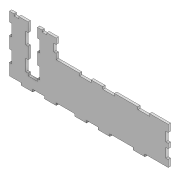
# Autodesk Inventor part: Frontal
Saved by Autodesk Inventor 2022 (Build 260153000, 153)
## iProperties
Created: 2022-06-21
Part Number: Frontal
Material: Generic
Document SubType Name: Modeling
Designer: ADMIN
Density: 1 g/cm^3
Appearance: Default
Author: ADMIN
Autodesk Inventor part; units mm, degrees
ref_plane "YZ Plane" through (0, 0, 0) normal (1, 0, 0) x (0, 1, 0)
ref_plane "XZ Plane" through (0, 0, 0) normal (0, 1, 0) x (-1, 0, 0)
ref_plane "XY Plane" through (0, 0, 0) normal (0, 0, 1) x (1, 0, 0)
sketch "Sketch1" plane through (0, 0, 0) normal (0, 0, 1) x (1, 0, 0)
  line L0 (-188.4506, 42.0684) -> (-148.4506, 42.0684)
  line L1 (-148.4506, 42.0684) -> (-148.4506, 2.0684)
  line L2 (-148.4506, 2.0684) -> (91.5494, 2.0684)
  line L3 (-198.4506, -77.9316) -> (91.5494, -77.9316)
  line L4 (91.5494, -77.9316) -> (91.5494, 2.0684)
  line L5 (-188.4506, -57.9316) -> (-208.4506, -57.9316)
  line L6 (-208.4506, -57.9316) -> (-208.4506, 42.0684)
  line L7 (-208.4506, 42.0684) -> (-248.4506, 42.0684)
  line L8 (-248.4506, 42.0684) -> (-248.4506, -77.9316)
  line L9 (-248.4506, -77.9316) -> (-198.4506, -77.9316)
  line L10 (-188.4506, -57.9316) -> (-188.4506, 42.0684)
  point P0 (0, 0)
  dimension "d2" = 80
  dimension "d3" = 40
  dimension "d23" = 40
  dimension "d24" = 20
  dimension "d26" = 20
  dimension "d27" = 120
  dimension "d28" = 120
  dimension "d58" = 280
  constraints: 22 end point, 3 perpendicular, 1 collinear, 1 horizontal, 1 vertical
  measures "d2" distance of L3.end L2.end
  measures "d3" distance of L0.start L0.end
  measures "d23" distance of L6.end L7.end
  measures "d24" distance of L5.start L5.end
  measures "d26" distance between parallel lines of L9 L5
  measures "d27" distance between parallel lines of L9 L7
  measures "d28" distance between parallel lines of L3 L0
  measures "d58" distance between parallel lines of L10 L4
extrude "Extrusion1" add sketch "Sketch1" along normal blind 5
sketch "Sketch2" plane through (0, 0, 5) normal (0, 0, 1) x (1, 0, 0)
  line L0 (91.5494, 2.0684) -> (-148.4506, 2.0684) projected
  line L1 (-148.4506, 2.0684) -> (-148.4506, 42.0684) projected
  line L2 (-148.4506, 42.0684) -> (-188.4506, 42.0684) projected
  line L3 (-248.4506, -77.9316) -> (91.5494, -77.9316) projected
  line L4 (91.5494, -77.9316) -> (91.5494, 2.0684) projected
  line L5 (91.5494, 2.0684) -> (-148.4506, 2.0684) projected
  line L6 (-98.4506, 2.0684) -> (-73.4506, 2.0684)
  line L7 (-73.4506, 2.0684) -> (-73.4506, -2.9316)
  line L8 (-73.4506, -2.9316) -> (-98.4506, -2.9316)
  line L9 (-98.4506, -2.9316) -> (-98.4506, 2.0684)
  line L10 (-48.4506, 2.0684) -> (-23.4506, 2.0684)
  line L11 (-23.4506, 2.0684) -> (-23.4506, -2.9316)
  line L12 (-23.4506, -2.9316) -> (-48.4506, -2.9316)
  line L13 (-48.4506, -2.9316) -> (-48.4506, 2.0684)
  line L14 (26.5494, 2.0684) -> (51.5494, 2.0684)
  line L15 (51.5494, 2.0684) -> (51.5494, -2.9316)
  line L16 (51.5494, -2.9316) -> (26.5494, -2.9316)
  line L17 (26.5494, -2.9316) -> (26.5494, 2.0684)
  line L18 (-148.4506, 42.0684) -> (-188.4506, 42.0684) projected
  line L19 (91.5494, -77.9316) -> (91.5494, 2.0684) projected
  line L20 (-73.4506, -7.9316) -> (-73.4506, -2.9316)
  line L21 (-98.4506, -2.9316) -> (-98.4506, -7.9316)
  line L22 (-23.4506, -7.9316) -> (-23.4506, -2.9316)
  line L23 (-48.4506, -2.9316) -> (-48.4506, -7.9316)
  line L24 (51.5494, -7.9316) -> (51.5494, -2.9316)
  line L25 (26.5494, -2.9316) -> (26.5494, -7.9316)
  line L26 (41.5494, -77.9316) -> (41.5494, -72.9316)
  line L27 (41.5494, -72.9316) -> (16.5494, -72.9316)
  line L28 (16.5494, -72.9316) -> (16.5494, -77.9316)
  line L29 (16.5494, -72.9316) -> (16.5494, -67.9316)
  line L30 (41.5494, -67.9316) -> (41.5494, -72.9316)
  line L31 (-188.4506, -57.9316) -> (-208.4506, -57.9316) projected
  line L32 (-208.4506, -57.9316) -> (-208.4506, 42.0684) projected
  line L33 (-208.4506, 42.0684) -> (-248.4506, 42.0684) projected
  line L34 (-248.4506, 42.0684) -> (-248.4506, -77.9316) projected
  line L35 (-188.4506, 42.0684) -> (-188.4506, -57.9316) projected
  line L36 (-208.4506, 42.0684) -> (-248.4506, 42.0684) projected
  line L37 (-238.4506, 42.0684) -> (-228.4506, 42.0684)
  line L38 (-228.4506, 42.0684) -> (-228.4506, 38.0682)
  line L39 (-228.4506, 38.0682) -> (-238.4506, 38.0682)
  line L40 (-238.4506, 38.0682) -> (-238.4506, 42.0684)
  line L41 (-148.4506, 42.0684) -> (-188.4506, 42.0684) projected
  line L42 (-178.4506, 42.0684) -> (-168.4506, 42.0684)
  line L43 (-168.4506, 42.0684) -> (-168.4506, 38.0682)
  line L44 (-168.4506, 38.0682) -> (-178.4506, 38.0682)
  line L45 (-178.4506, 38.0682) -> (-178.4506, 42.0684)
  line L46 (-248.4506, 42.0684) -> (-248.4506, -77.9316) projected
  line L47 (-248.4506, 22.0684) -> (-243.4506, 22.0684)
  line L48 (-243.4506, 22.0684) -> (-243.4506, -2.9316)
  line L49 (-243.4506, -2.9316) -> (-248.4506, -2.9316)
  line L50 (-248.4506, -2.9316) -> (-248.4506, 22.0684)
  line L51 (-248.4506, -52.9316) -> (-243.4506, -52.9316)
  line L52 (-243.4506, -52.9316) -> (-243.4506, -27.9316)
  line L53 (-243.4506, -27.9316) -> (-248.4506, -27.9316)
  line L54 (-248.4506, -27.9316) -> (-248.4506, -52.9316)
  line L55 (-188.4506, 42.0684) -> (-188.4506, -57.9316) projected
  line L56 (-188.4506, 22.0684) -> (-183.4506, 22.0684)
  line L57 (-183.4506, 22.0684) -> (-183.4506, -2.9316)
  line L58 (-183.4506, -2.9316) -> (-188.4506, -2.9316)
  line L59 (-188.4506, -2.9316) -> (-188.4506, 22.0684)
  line L60 (-188.4506, -27.9316) -> (-183.4506, -27.9316)
  line L61 (-183.4506, -27.9316) -> (-183.4506, -52.9316)
  line L62 (-183.4506, -52.9316) -> (-188.4506, -52.9316)
  line L63 (-188.4506, -52.9316) -> (-188.4506, -27.9316)
  line L64 (-208.4506, -57.9316) -> (-208.4506, 42.0684) projected
  line L65 (-208.4506, 22.0684) -> (-213.4506, 22.0684)
  line L66 (-213.4506, 22.0684) -> (-213.4506, -2.9316)
  line L67 (-213.4506, -2.9316) -> (-208.4506, -2.9316)
  line L68 (-208.4506, -2.9316) -> (-208.4506, 22.0684)
  line L69 (-208.4506, -52.9316) -> (-213.4506, -52.9316)
  line L70 (-213.4506, -52.9316) -> (-213.4506, -27.9316)
  line L71 (-213.4506, -27.9316) -> (-208.4506, -27.9316)
  line L72 (-208.4506, -27.9316) -> (-208.4506, -52.9316)
  line L73 (-148.4506, 2.0684) -> (-148.4506, 42.0684) projected
  line L74 (-148.4506, 30.0684) -> (-153.4506, 30.0684)
  line L75 (-153.4506, 30.0684) -> (-153.4506, 14.0684)
  line L76 (-153.4506, 14.0684) -> (-148.4506, 14.0684)
  line L77 (-148.4506, 14.0684) -> (-148.4506, 30.0684)
  line L78 (-248.4506, -77.9316) -> (91.5494, -77.9316) projected
  line L79 (-223.4506, -77.9316) -> (-198.4506, -77.9316)
  line L80 (-198.4506, -77.9316) -> (-198.4506, -72.9316)
  line L81 (-198.4506, -72.9316) -> (-223.4506, -72.9316)
  line L82 (-223.4506, -72.9316) -> (-223.4506, -77.9316)
  line L83 (-173.4506, -77.9316) -> (-148.4506, -77.9316)
  line L84 (-148.4506, -77.9316) -> (-148.4506, -72.9316)
  line L85 (-148.4506, -72.9316) -> (-173.4506, -72.9316)
  line L86 (-173.4506, -72.9316) -> (-173.4506, -77.9316)
  line L87 (-108.4506, -77.9316) -> (-83.4506, -77.9316)
  line L88 (-83.4506, -77.9316) -> (-83.4506, -72.9316)
  line L89 (-83.4506, -72.9316) -> (-108.4506, -72.9316)
  line L90 (-108.4506, -72.9316) -> (-108.4506, -77.9316)
  line L91 (-58.4506, -77.9316) -> (-33.4506, -77.9316)
  line L92 (-33.4506, -77.9316) -> (-33.4506, -72.9316)
  line L93 (-33.4506, -72.9316) -> (-58.4506, -72.9316)
  line L94 (-58.4506, -72.9316) -> (-58.4506, -77.9316)
  line L95 (91.5494, -12.9316) -> (86.5494, -12.9316)
  line L96 (86.5494, -12.9316) -> (86.5494, -32.9316)
  line L97 (86.5494, -32.9316) -> (91.5494, -32.9316)
  line L98 (91.5494, -32.9316) -> (91.5494, -12.9316)
  line L99 (91.5494, -62.9316) -> (86.5494, -62.9316)
  line L100 (86.5494, -62.9316) -> (86.5494, -42.9316)
  line L101 (86.5494, -42.9316) -> (91.5494, -42.9316)
  line L102 (91.5494, -42.9316) -> (91.5494, -62.9316)
  point P0 (0, 0)
  point P1 (0, -75.8632)
  point P2 (91.5494, -32.9316)
  point P3 (91.5494, -12.9316)
  point P4 (51.5494, 2.0684)
  point P5 (26.5494, 2.0684)
  point P6 (-23.4506, 2.0684)
  point P7 (-48.4506, 2.0684)
  point P8 (-73.4506, 2.0684)
  point P9 (-98.4506, 2.0684)
  point P10 (-188.4506, -27.9316)
  point P11 (-148.4506, 14.0684)
  point P12 (-148.4506, 30.0684)
  point P13 (-188.4506, -2.9316)
  point P14 (-168.4506, 42.0684)
  point P15 (-178.4506, 42.0684)
  point P16 (-208.4506, -2.9316)
  dimension "d6" = 25
  dimension "d7" = 5
  dimension "d8" = 25
  dimension "d9" = 25
  dimension "d10" = 5
  dimension "d20" = 40
  dimension "d21" = 50
  dimension "d22" = 25
  dimension "d29" = 5
  dimension "d30" = 25
  dimension "d31" = 5
  dimension "d32" = 25
  dimension "d33" = 25
  dimension "d34" = 25
  dimension "d35" = 5
  dimension "d36" = 5
  dimension "d37" = 5
  dimension "d38" = 16
  dimension "d39" = 12
  dimension "d40" = 25
  dimension "d41" = 5
  dimension "d42" = 25
  dimension "d44" = 25
  dimension "d45" = 25
  dimension "d46" = 5
  dimension "d47" = 5
  dimension "d48" = 20
  dimension "d49" = 20
  dimension "d50" = 10
  dimension "d51" = 15
  dimension "d54" = 10
  dimension "d55" = 10
  dimension "d56" = 10
  dimension "d57" = 10
  constraints: 166 end point, 36 parallel, 24 point on line, 18 horizontal, 18 perpendicular, 6 symmetric about line
  measures "d6" distance of L7.end L8.end
  measures "d7" distance of L6.end L7.end
  measures "d8" distance of L11.end L12.end
  measures "d9" distance of L15.end L16.end
  measures "d10" distance of L14.end L15.end
  measures "d20" distance between parallel lines of L4 L15
  measures "d21" distance between parallel lines of L17 L11
  measures "d22" distance between parallel lines of L13 L7
  measures "d29" distance of L48.end L49.end
  measures "d30" distance of L47.end L48.end
  measures "d31" distance of L53.end L52.end
  measures "d32" distance of L52.end L51.end
  measures "d33" distance between parallel lines of L53 L49
  measures "d34" distance between parallel lines of L3 L51
  measures "d35" distance of L57.end L58.end
  measures "d36" distance of L67.end L66.end
  measures "d37" distance of L76.end L75.end
  measures "d38" distance of L75.end L74.end
  measures "d39" distance between parallel lines of L74 L2
  measures "d40" distance of L81.end L80.end
  measures "d41" distance of L80.end L79.end
  measures "d42" distance of L85.end L84.end
  measures "d44" distance between parallel lines of L80 L86
  measures "d45" distance between parallel lines of L34 L82
  measures "d46" distance of L88.end L87.end
  measures "d47" distance of L97.end L96.end
  measures "d48" distance of L96.end L95.end
  measures "d49" distance of L99.end L100.end
  measures "d50" distance between parallel lines of L101 L97
  measures "d51" distance between parallel lines of L3 L99
  measures "d54" distance between parallel lines of L35 L45
  measures "d55" distance of L43.end L44.end
  measures "d56" distance of L38.end L39.end
  measures "d57" distance between parallel lines of L34 L40
extrude "Extrusion2" cut sketch "Sketch2" against normal blind 5 contours L15 L16 L17 L0 | L4 L97 L96 L95 | L11 L12 L13 L0 | L4 L99 L100 L101 | L7 L8 L9 L0 | L3 L28 L27 L26 | L76 L75 L74 L1 | L3 L94 L93 L92 | L3 L90 L89 L88 | L43 L44 L45 L2 | L3 L86 L85 L84 | L56 L57 L58 L35 | L3 L82 L81 L80 | L60 L61 L62 L35 | L34 L53 L52 L51 | L34 L47 L48 L49 | L69 L70 L71 L32 | L67 L66 L65 L32 | L33 L38 L39 L40
sketch "Sketch3" plane through (0, 0, 5) normal (0, 0, 1) x (1, 0, 0)
  line L0 (-178.4506, 38.0682) -> (-178.4506, 42.0684) projected
  line L1 (-178.4506, 42.0684) -> (-188.4506, 42.0684) projected
  line L2 (-188.4506, 42.0684) -> (-188.4506, 22.0684) projected
  line L3 (-188.4506, 22.0684) -> (-183.4506, 22.0684) projected
  line L4 (-183.4506, 22.0684) -> (-183.4506, -2.9316) projected
  line L5 (-183.4506, -2.9316) -> (-188.4506, -2.9316) projected
  line L6 (-188.4506, -2.9316) -> (-188.4506, -27.9316) projected
  line L7 (-188.4506, -27.9316) -> (-183.4506, -27.9316) projected
  line L8 (-183.4506, -27.9316) -> (-183.4506, -52.9316) projected
  line L9 (-183.4506, -52.9316) -> (-188.4506, -52.9316) projected
  line L10 (-188.4506, -52.9316) -> (-188.4506, -57.9316) projected
  line L11 (-188.4506, -57.9316) -> (-208.4506, -57.9316) projected
  line L12 (-208.4506, -57.9316) -> (-208.4506, -52.9316) projected
  line L13 (-208.4506, -52.9316) -> (-213.4506, -52.9316) projected
  line L14 (-213.4506, -52.9316) -> (-213.4506, -27.9316) projected
  line L15 (-213.4506, -27.9316) -> (-208.4506, -27.9316) projected
  line L16 (-208.4506, -27.9316) -> (-208.4506, -2.9316) projected
  line L17 (-208.4506, -2.9316) -> (-213.4506, -2.9316) projected
  line L18 (-213.4506, -2.9316) -> (-213.4506, 22.0684) projected
  line L19 (-213.4506, 22.0684) -> (-208.4506, 22.0684) projected
  line L20 (-208.4506, 22.0684) -> (-208.4506, 42.0684) projected
  line L21 (-208.4506, 42.0684) -> (-228.4506, 42.0684) projected
  line L22 (-228.4506, 42.0684) -> (-228.4506, 38.0682) projected
  line L23 (-228.4506, 38.0682) -> (-238.4506, 38.0682) projected
  line L24 (-238.4506, 38.0682) -> (-238.4506, 42.0684) projected
  line L25 (-238.4506, 42.0684) -> (-248.4506, 42.0684) projected
  line L26 (-248.4506, 42.0684) -> (-248.4506, 22.0684) projected
  line L27 (-248.4506, 22.0684) -> (-243.4506, 22.0684) projected
  line L28 (-243.4506, 22.0684) -> (-243.4506, -2.9316) projected
  line L29 (-243.4506, -2.9316) -> (-248.4506, -2.9316) projected
  line L30 (-248.4506, -2.9316) -> (-248.4506, -27.9316) projected
  line L31 (-248.4506, -27.9316) -> (-243.4506, -27.9316) projected
  line L32 (-243.4506, -27.9316) -> (-243.4506, -52.9316) projected
  line L33 (-243.4506, -52.9316) -> (-248.4506, -52.9316) projected
  line L34 (-248.4506, -52.9316) -> (-248.4506, -77.9316) projected
  line L35 (-248.4506, -77.9316) -> (-223.4506, -77.9316) projected
  line L36 (-223.4506, -77.9316) -> (-223.4506, -72.9316) projected
  line L37 (-223.4506, -72.9316) -> (-198.4506, -72.9316) projected
  line L38 (-198.4506, -72.9316) -> (-198.4506, -77.9316) projected
  line L39 (-198.4506, -77.9316) -> (-173.4506, -77.9316) projected
  line L40 (-173.4506, -77.9316) -> (-173.4506, -72.9316) projected
  line L41 (-173.4506, -72.9316) -> (-148.4506, -72.9316) projected
  line L42 (-148.4506, -72.9316) -> (-148.4506, -77.9316) projected
  line L43 (-148.4506, -77.9316) -> (-108.4506, -77.9316) projected
  line L44 (-108.4506, -77.9316) -> (-108.4506, -72.9316) projected
  line L45 (-108.4506, -72.9316) -> (-83.4506, -72.9316) projected
  line L46 (-83.4506, -72.9316) -> (-83.4506, -77.9316) projected
  line L47 (-83.4506, -77.9316) -> (-58.4506, -77.9316) projected
  line L48 (-58.4506, -77.9316) -> (-58.4506, -72.9316) projected
  line L49 (-58.4506, -72.9316) -> (-33.4506, -72.9316) projected
  line L50 (-33.4506, -72.9316) -> (-33.4506, -77.9316) projected
  line L51 (-33.4506, -77.9316) -> (16.5494, -77.9316) projected
  line L52 (16.5494, -77.9316) -> (16.5494, -72.9316) projected
  line L53 (16.5494, -72.9316) -> (41.5494, -72.9316) projected
  line L54 (41.5494, -72.9316) -> (41.5494, -77.9316) projected
  line L55 (41.5494, -77.9316) -> (91.5494, -77.9316) projected
  line L56 (91.5494, -77.9316) -> (91.5494, -62.9316) projected
  line L57 (91.5494, -62.9316) -> (86.5494, -62.9316) projected
  line L58 (86.5494, -62.9316) -> (86.5494, -42.9316) projected
  line L59 (86.5494, -42.9316) -> (91.5494, -42.9316) projected
  line L60 (91.5494, -42.9316) -> (91.5494, -32.9316) projected
  line L61 (91.5494, -32.9316) -> (86.5494, -32.9316) projected
  line L62 (86.5494, -32.9316) -> (86.5494, -12.9316) projected
  line L63 (86.5494, -12.9316) -> (91.5494, -12.9316) projected
  line L64 (91.5494, -12.9316) -> (91.5494, 2.0684) projected
  line L65 (91.5494, 2.0684) -> (51.5494, 2.0684) projected
  line L66 (51.5494, 2.0684) -> (51.5494, -2.9316) projected
  line L67 (51.5494, -2.9316) -> (26.5494, -2.9316) projected
  line L68 (26.5494, -2.9316) -> (26.5494, 2.0684) projected
  line L69 (26.5494, 2.0684) -> (-23.4506, 2.0684) projected
  line L70 (-23.4506, 2.0684) -> (-23.4506, -2.9316) projected
  line L71 (-23.4506, -2.9316) -> (-48.4506, -2.9316) projected
  line L72 (-48.4506, -2.9316) -> (-48.4506, 2.0684) projected
  line L73 (-48.4506, 2.0684) -> (-73.4506, 2.0684) projected
  line L74 (-73.4506, 2.0684) -> (-73.4506, -2.9316) projected
  line L75 (-73.4506, -2.9316) -> (-98.4506, -2.9316) projected
  line L76 (-98.4506, -2.9316) -> (-98.4506, 2.0684) projected
  line L77 (-98.4506, 2.0684) -> (-148.4506, 2.0684) projected
  line L78 (-148.4506, 2.0684) -> (-148.4506, 14.0684) projected
  line L79 (-148.4506, 14.0684) -> (-153.4506, 14.0684) projected
  line L80 (-153.4506, 14.0684) -> (-153.4506, 30.0684) projected
  line L81 (-153.4506, 30.0684) -> (-148.4506, 30.0684) projected
  line L82 (-148.4506, 30.0684) -> (-148.4506, 42.0684) projected
  line L83 (-148.4506, 42.0684) -> (-168.4506, 42.0684) projected
  line L84 (-168.4506, 42.0684) -> (-168.4506, 38.0682) projected
  line L85 (-168.4506, 38.0682) -> (-178.4506, 38.0682) projected
  line L86 (-223.4506, -72.9316) -> (-198.4506, -72.9316)
  line L87 (-198.4506, -72.9316) -> (-198.4506, -82.9316)
  line L88 (-198.4506, -82.9316) -> (-223.4506, -82.9316)
  line L89 (-223.4506, -82.9316) -> (-223.4506, -72.9316)
  line L90 (-148.4506, -72.9316) -> (-173.4506, -72.9316) projected
  line L91 (-173.4506, -72.9316) -> (-148.4506, -72.9316)
  line L92 (-148.4506, -72.9316) -> (-148.4506, -82.9316)
  line L93 (-148.4506, -82.9316) -> (-173.4506, -82.9316)
  line L94 (-173.4506, -82.9316) -> (-173.4506, -72.9316)
  line L95 (-108.4506, -72.9316) -> (-83.4506, -72.9316)
  line L96 (-83.4506, -72.9316) -> (-83.4506, -82.9316)
  line L97 (-83.4506, -82.9316) -> (-108.4506, -82.9316)
  line L98 (-108.4506, -82.9316) -> (-108.4506, -72.9316)
  line L99 (-33.4506, -72.9316) -> (-58.4506, -72.9316) projected
  line L100 (-58.4506, -72.9316) -> (-33.4506, -72.9316)
  line L101 (-33.4506, -72.9316) -> (-33.4506, -82.9316)
  line L102 (-33.4506, -82.9316) -> (-58.4506, -82.9316)
  line L103 (-58.4506, -82.9316) -> (-58.4506, -72.9316)
  line L104 (16.5494, -72.9316) -> (41.5494, -72.9316) projected
  line L105 (16.5494, -72.9316) -> (41.5494, -72.9316)
  line L106 (41.5494, -72.9316) -> (41.5494, -82.9316)
  line L107 (41.5494, -82.9316) -> (16.5494, -82.9316)
  line L108 (16.5494, -82.9316) -> (16.5494, -72.9316)
  point P0 (0, 0)
  dimension "d59" = 10
  dimension "d60" = 10
  dimension "d61" = 10
  dimension "d62" = 10
  dimension "d63" = 10
  constraints: 40 end point, 10 parallel, 5 horizontal, 5 perpendicular
  measures "d59" distance of L86.end L87.end
  measures "d60" distance of L91.end L92.end
  measures "d61" distance of L95.end L96.end
  measures "d62" distance of L100.end L101.end
  measures "d63" distance of L105.end L106.end
extrude "Extrusion3" add sketch "Sketch3" against normal blind 5 contours L106 L107 L108 L52 L53 L54 | L101 L102 L103 L48 L49 L50 | L36 L37 L38 L87 L88 L89 | L96 L97 L98 L44 L45 L46 | L40 L41 L42 L92 L93 L94
body "Solid1"
